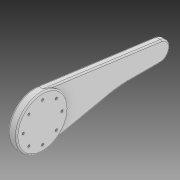
# Autodesk Inventor part: TestArm
Saved by Autodesk Inventor 2020 (Build 240168000, 168)
## iProperties
Created: 2021-04-06
Part Number: TestArm
Material: Generic
Document SubType Name: Modeling
Designer: DDeGo
Density: 1 g/cm^3
Appearance: Default
Author: DDeGo
Autodesk Inventor part; units mm, degrees
ref_plane "YZ Plane" through (0, 0, 0) normal (1, 0, 0) x (0, 1, 0)
ref_plane "XZ Plane" through (0, 0, 0) normal (0, 1, 0) x (-1, 0, 0)
ref_plane "XY Plane" through (0, 0, 0) normal (0, 0, 1) x (1, 0, 0)
sketch "Sketch1" plane through (0, 0, 0) normal (1, 0, 0) x (0, 1, 0)
  circle A0 centre (0, 0) radius 30 construction
  arc A1 (39.633087, -5.405405) -> (-39.117675, -8.35509) centre (0, 0) ccw
  arc A2 (-15, -185) -> (14.862408, -187.027027) centre (0, -185) ccw
  line L0 (39.633087, -5.405405) -> (14.862408, -187.027027)
  line L1 (0, 0) -> (0, -185) construction
  line L2 (74.717365, 40) -> (-69.808973, 40) construction
  line L3 (-69.808973, 40) -> (-69.808973, -200) construction
  line L4 (-69.808973, -200) -> (74.717365, -200) construction
  line L5 (74.717365, -200) -> (74.717365, 40) construction
  line L6 (-15, -185) -> (-15, -135)
  line L7 (-17.867558, -107.845957) -> (-39.117675, -8.35509)
  arc A3 (-15, -135) -> (-17.867558, -107.845957) centre (-145, -135) ccw
  circle A4 centre (0, -30) radius 1.75
  circle A5 centre (21.213203, -21.213203) radius 1.75
  circle A6 centre (30, 0) radius 1.75
  circle A7 centre (21.213203, 21.213203) radius 1.75
  circle A8 centre (0, 30) radius 1.75
  circle A9 centre (-21.213203, 21.213203) radius 1.75
  circle A10 centre (-30, 0) radius 1.75
  circle A11 centre (-21.213203, -21.213203) radius 1.75
  dimension "d0" = 60
  dimension "d1" = 80
  dimension "d2" = 30
  dimension "d3" = 240
  dimension "d4" = 130
  dimension "d5" = 50
  dimension "d6" = 3.5
  dimension "d9" = 360
  dimension "d15" = 185
  constraints: 16 end point, 11 centre point, 8 tangent, 6 point on circle, 2 coincident, 2 parallel, 2 vertical, 1 horizontal, 1 perpendicular, 1 point on line, 1 vertical alignment, 19 other
  measures "d1" diameter of A1
  measures "d2" diameter of A2
  measures "d3" distance between parallel lines of L2 L4
  measures "d4" radius of A3
  measures "d5" distance of L6.start L6.end
  measures "d6" diameter of A4
  measures "d15" distance of L1.start L1.end
extrude "Extrusion1" add sketch "Sketch1" along normal blind 10
sketch "Sketch2" plane through (10, 0, 0) normal (1, 0, 0) x (0, 0, -1)
  arc A0 (135, -15) -> (107.845957, -17.867558) centre (135, -145) ccw
  line L0 (135, -15) -> (185, -15)
  arc A1 (185, -15) -> (187.027027, 14.862408) centre (185, 0) ccw
  line L1 (187.027027, 14.862408) -> (5.405405, 39.633087)
  arc A2 (5.405405, 39.633087) -> (8.35509, -39.117675) centre (0, 0) ccw
  line L2 (8.35509, -39.117675) -> (107.845957, -17.867558)
  circle A3 centre (30, 0) radius 1.75
  circle A4 centre (21.213203, -21.213203) radius 1.75
  circle A5 centre (0, -30) radius 1.75
  circle A6 centre (-21.213203, -21.213203) radius 1.75
  circle A7 centre (-30, 0) radius 1.75
  circle A8 centre (-21.213203, 21.213203) radius 1.75
  circle A9 centre (0, 30) radius 1.75
  circle A10 centre (21.213203, 21.213203) radius 1.75
  arc A11 (5.405405, 39.633087) -> (8.35509, -39.117675) centre (0, 0) ccw
  circle A12 centre (0, 0) radius 40
  point P0 (5.405405, 39.633087)
  constraints: 1 coincident, 3 other
extrude "Extrusion2" add sketch "Sketch2" along normal blind 3 contours A2 A12
fillet "Fillet1" radius 2 12 edges at (10, -1.0158, -199.9656) (10, -15, -160) (10, -15.7189, -121.3475) (10, -28.4926, -58.1005) (10, 27.2477, -96.2162) (0, -1.4972, 39.972) (0, -28.4926, -58.1005) (0, -15.7189, -121.3475) (0, -15, -160) (0, -1.0158, -199.9656) (0, 27.2477, -96.2162) (13, 39.1177, 8.3551)
body "Solid1"
